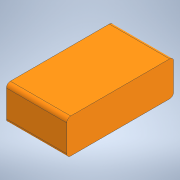
# Autodesk Inventor part: Battery[54x30_5x17_5]
Saved by Autodesk Inventor 2021 (Build 250183000, 183)
## iProperties
Created: 2021-02-15
Part Number: Battery[54x30_5x17_5]
Material: Generic
Document SubType Name: Modeling
Designer: ermoz
Density: 1 g/cm^3
Appearance: Default
Author: ermoz
Autodesk Inventor part; units mm, degrees
ref_plane "YZ Plane" through (0, 0, 0) normal (1, 0, 0) x (0, 1, 0)
ref_plane "XZ Plane" through (0, 0, 0) normal (0, 1, 0) x (-1, 0, 0)
ref_plane "XY Plane" through (0, 0, 0) normal (0, 0, 1) x (1, 0, 0)
sketch "Sketch1" plane through (0, 0, 0) normal (0, 1, 0) x (-1, 0, 0)
  line L0 (-15.25, 27) -> (15.25, 27)
  line L1 (15.25, 27) -> (15.25, -27)
  line L2 (15.25, -27) -> (-15.25, -27)
  line L3 (-15.25, -27) -> (-15.25, 27)
  line L4 (-15.25, 27) -> (15.25, -27) construction
  line L5 (15.25, 27) -> (-15.25, -27) construction
  point P0 (0, 0)
  dimension "d0" = 30.5
  dimension "d1" = 54
  constraints: 12 end point, 2 midpoint, 2 parallel, 1 horizontal, 1 perpendicular
  measures "d0" distance of L1.end L2.end
  measures "d1" distance of L0.end L1.end
extrude "Extrusion1" add sketch "Sketch1" along normal blind 17.5
fillet "Fillet1" radius 2 4 edges at (0, 17.5, -27) (0, 0, -27) (0, 17.5, 27) (0, 0, 27)
body "Solid1"
